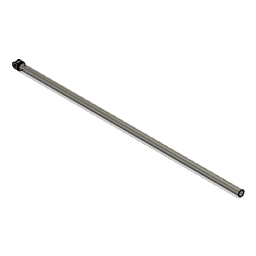
Tube 38 - IGTE 204894 (Autodesk Fusion 360 design; units mm, degrees)
Autodesk Fusion 360 part; units mm, degrees
note: some values were not read from the file. Chosen so that the rebuilt part matches the saved one: which pieces of a blend or face edit are solid.
sketch "Sketch1" plane through (0, 0, 0) normal (0, 0, 1) x (1, 0, 0)
  circle A0 centre (0, 0) radius 6
  line L0 (0, 0) -> (0, 49.4759) construction
  line L1 (0, 0) -> (0, -54.6862) construction
  arc A1 (0, 18) -> (0, -18) centre (0, 0) ccw
  line L2 (0, 18) -> (25, 18)
  line L3 (0, -18) -> (25, -18)
  line L4 (25, 18) -> (25, -18)
  dimension "d1" = 36
  dimension "d2" = 12
  dimension "d4" = 25
  dimension "d5" = 25
  constraint coincident A0.centre L0.start
  constraint vertical L0
  constraint parallel L0 L1
  constraint coincident L1 A1.end
  constraint coincident L0 A1.start
  constraint perpendicular L3 L4
  measures "d1" diameter of A1
  measures "d2" diameter of A0
  measures "d4" distance of A1.start L2.end
  measures "d5" distance of A1.end L3.end
extrude "Extrude1" add sketch "Sketch1" along normal mid plane 30
sketch "Sketch2" plane through (25, 0, 0) normal (1, 0, 0) x (0, 0, -1)
  line L0 (15, 18) -> (-15, 18)
  line L1 (-15, 18) -> (-15, -18)
  line L2 (-15, -18) -> (15, -18)
  line L3 (15, -18) -> (15, 18)
  circle A0 centre (0, 0) radius 19
  circle A1 centre (0, 0) radius 17
  dimension "d8" = 38
  dimension "d9" = 34
  constraint coincident A0.centre A1.centre
  measures "d8" diameter of A0
  measures "d9" diameter of A1
extrude "Extrude2" add sketch "Sketch2" along normal blind 1500 contours L0 L1 L3 A0 A1 | L0 A0 | L3 A0 A1 | L1 A0 A1 | L1 L2 L3 A0 A1 | L2 A0
ref_plane "WorkPlane1" through (25, 0, 0) normal (1, 0, 0) x (0, 1, 0)
sketch "Sketch3" plane through (25, 0, 0) normal (1, 0, 0) x (0, 0, -1)
  line L0 (-6.0828, 18) -> (-15, 18)
  line L1 (-15, 11.6619) -> (-15, 18)
  line L2 (15, 18) -> (6.0828, 18)
  line L3 (15, 18) -> (15, 11.6619)
  line L4 (-6.0828, -18) -> (-15, -18)
  line L5 (-15, -18) -> (-15, -11.6619)
  line L6 (15, -18) -> (6.0828, -18)
  line L7 (15, -11.6619) -> (15, -18)
  circle A0 centre (0, 0) radius 23.4307
  constraint coincident A0.centre origin
  constraint coincident L4.end A0
extrude "Extrude3" add sketch "Sketch3" along normal mid plane 5
fillet "Fillet1" radius 5 4 edges at (22.5, 18, 0) (22.5, 0, 15) (22.5, -18, 0) (22.5, 0, -15)
sketch "Sketch4" plane through (0, 0, 0) normal (0, 1, 0) x (1, 0, 0)
  line L0 (0, 0) -> (50, 0) construction
  circle A0 centre (50, 0) radius 2.5
  dimension "d16" = 50
  dimension "d17" = 5
  constraint coincident L0.start origin
  constraint coincident L0.end A0.centre
  measures "d16" distance of L0.start L0.end
  measures "d17" diameter of A0
extrude "Extrude4" cut sketch "Sketch4" along normal through all and the other way through all
sketch "Sketch5" plane through (0, 0, 0) normal (0, 0, 1) x (1, 0, 0)
  line L0 (0, 0) -> (50, 0) construction
  circle A0 centre (50, 0) radius 2.5
  dimension "d20" = 50
  dimension "d21" = 5
  constraint coincident L0.start origin
  constraint coincident L0.end A0.centre
  measures "d20" distance of L0.start L0.end
  measures "d21" diameter of A0
extrude "Extrude5" cut sketch "Sketch5" along normal through all and the other way through all
equation "d1 = ( 18 * 2 ) * 1 mm"
